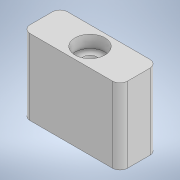
# Autodesk Inventor part: Soporte placa A1 - A2
Saved by Autodesk Inventor 2020 (Build 240168000, 168)
## iProperties
Created: 2020-05-18
Part Number: Soporte placa A1 - A2
Material: Genérico
Document SubType Name: Modeling
Designer: javic
Density: 1 g/cm^3
Appearance: Valor por defecto
Author: javic
Autodesk Inventor part; units mm, degrees
ref_plane "YZ Plane" through (0, 0, 0) normal (1, 0, 0) x (0, 1, 0)
ref_plane "XZ Plane" through (0, 0, 0) normal (0, 1, 0) x (-1, 0, 0)
ref_plane "XY Plane" through (0, 0, 0) normal (0, 0, 1) x (1, 0, 0)
sketch "Boceto1" plane through (0, 0, 0) normal (0, 1, 0) x (-1, 0, 0)
  line L0 (0, 0) -> (0, -5)
  line L1 (0, -5) -> (13, -5)
  line L2 (13, -5) -> (13, 0)
  line L3 (13, 0) -> (0, 0)
  circle A0 centre (6.5, -2.5) radius 0.9
  dimension "d0" = 5
  dimension "d1" = 13
  dimension "d2" = 1.8
  constraints: 8 end point, 3 perpendicular, 1 centre point, 1 vertical
  measures "d0" distance of L0.start L0.end
  measures "d1" distance of L0.end L1.end
  measures "d2" diameter of A0
extrude "Extrusión1" add sketch "Boceto1" along normal blind 10.06
sketch "Boceto2" plane through (0, 10.06, 0) normal (0, 1, 0) x (1, 0, 0)
  circle A0 centre (-6.5, 2.5) radius 0.9 projected
  point P0 (0, 0)
  constraints: 3 coincident
hole "Agujero1" at (-6.5, 10.06, -2.5) direction (0, -1, 0) diameter 4 depth 1.65
fillet "Empalme1" radius 1 4 edges at (0, 5.03, 0) (0, 5.03, -5) (-13, 5.03, 0) (-13, 5.03, -5)
